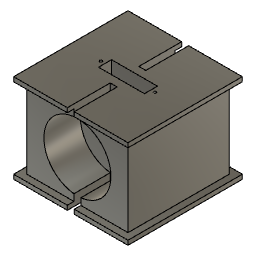
TWO MAG BODY 3x1.5 v01 (Autodesk Fusion 360 design; units mm, degrees)
Autodesk Fusion 360 part; units mm, degrees
note: some values were not read from the file. Set by a fixed rule: which sketch regions a step uses.
sketch "Sketch1" plane through (0, 0, 0) normal (0, 0, 1) x (1, 0, 0)
  line L0 (-30.48, 114.973) -> (86.36, 114.973)
  line L1 (86.36, 114.973) -> (86.36, -1.867)
  line L2 (86.36, -1.867) -> (-30.48, -1.867)
  line L3 (-30.48, -1.867) -> (-30.48, 114.973)
  line L4 (1.4449, 64.0587) -> (54.4449, 64.0587)
  line L5 (54.4449, 64.0587) -> (54.4449, 49.0587)
  line L6 (54.4449, 49.0587) -> (1.4449, 49.0587)
  line L7 (1.4449, 49.0587) -> (1.4449, 64.0587)
  line L8 (23.9405, 114.973) -> (31.9405, 114.973)
  line L9 (31.9405, 114.973) -> (31.9405, 73.063)
  line L10 (31.9405, 73.063) -> (23.9405, 73.063)
  line L11 (23.9405, 73.063) -> (23.9405, 114.973)
  line L12 (23.9405, -1.867) -> (31.9405, -1.867)
  line L13 (31.9405, -1.867) -> (31.9405, 40.043)
  line L14 (31.9405, 40.043) -> (23.9405, 40.043)
  line L15 (23.9405, 40.043) -> (23.9405, -1.867)
  dimension "d1" = 116.84
  dimension "d2" = 116.84
  dimension "d3" = 15
  dimension "d4" = 53
  dimension "d5" = 31.9151
  dimension "d8" = 50.9143
  dimension "d9" = 8
  dimension "d10" = 54.4195
  dimension "d11" = 41.91
  dimension "d12" = 41.91
  dimension "d13" = 54.4195
  dimension "d14" = 8
  constraint horizontal L0
  constraint vertical L1
  constraint horizontal L2
  constraint vertical L3
  constraint horizontal L4
  constraint vertical L5
  constraint horizontal L6
  constraint vertical L7
  constraint horizontal L8
  constraint vertical L9
  constraint horizontal L10
  constraint vertical L11
  constraint coincident L0 L8.start
  constraint horizontal L12
  constraint vertical L13
  constraint horizontal L14
  constraint vertical L15
  constraint coincident L2 L12.start
  measures "d1" distance of L0.end L1.end
  measures "d2" distance of L0.start L0.end
  measures "d3" distance of L4.end L5.end
  measures "d4" distance of L5.end L6.end
  measures "d5" distance of L1 L5
  measures "d8" distance of L0 L4
  measures "d9" distance of L13 L15
  measures "d10" distance of L1 L13
  measures "d11" distance of L12.end L13.end
  measures "d12" distance of L8.end L9.end
  measures "d13" distance of L1 L9
  measures "d14" distance of L9.end L10.end
extrude "Extrude1" add sketch "Sketch1" along normal blind 102.616 contours L0 L1 L2 L3 L9 L10 L11 L13 L14 L15
sketch "Sketch2" plane through (0, -1.867, 0) normal (0, -1, 0) x (1, 0, 0)
  line L0 (-30.48, 0) -> (23.9405, 0)
  line L1 (23.9405, 0) -> (23.9405, 102.616)
  line L2 (23.9405, 102.616) -> (-30.48, 102.616)
  line L3 (-30.48, 102.616) -> (-30.48, 0)
  circle A0 centre (27.94, 51.308) radius 38.735
  dimension "d17" = 77.47
  dimension "d18" = 51.308
  dimension "d19" = 58.42
  measures "d17" diameter of A0
  measures "d18" distance of L2 A0.centre
  measures "d19" distance of L3 A0.centre
extrude "Extrude2" cut sketch "Sketch2" against normal blind 42.037 contours L1 A0 | L1 A0
sketch "Sketch3" plane through (0, 114.973, 0) normal (0, 1, 0) x (-1, 0, 0)
  line L0 (-23.9405, 0) -> (30.48, 0)
  line L1 (30.48, 0) -> (30.48, 102.616)
  line L2 (30.48, 102.616) -> (-23.9405, 102.616)
  line L3 (-23.9405, 102.616) -> (-23.9405, 0)
  circle A0 centre (-27.94, 51.308) radius 38.735
  dimension "d22" = 77.47
  dimension "d23" = 58.42
  dimension "d24" = 51.308
  measures "d22" diameter of A0
  measures "d23" distance of L1 A0.centre
  measures "d24" distance of L2 A0.centre
extrude "Extrude3" cut sketch "Sketch3" against normal blind 42.037 contours L3 A0 | L3 A0
sketch "Sketch5" plane through (0, -1.867, 0) normal (0, -1, 0) x (1, 0, 0)
  arc A0 (31.9405, 12.7801) -> (31.9405, 89.8359) centre (27.94, 51.308) ccw
  line L0 (31.9405, 12.7801) -> (31.9405, 0)
  line L1 (31.9405, 0) -> (86.36, 0)
  line L2 (86.36, 0) -> (86.36, 102.616)
  line L3 (86.36, 102.616) -> (31.9405, 102.616)
  line L4 (31.9405, 102.616) -> (31.9405, 89.8359)
  line L5 (86.36, 102.616) -> (86.36, 97.536)
  line L6 (-30.48, 97.536) -> (-30.48, 102.616)
  line L7 (-30.48, 5.08) -> (-30.48, 0)
  line L8 (86.36, 0) -> (86.36, 5.08)
  line L9 (31.9405, 102.616) -> (31.9405, 97.536)
  line L10 (23.9405, 102.616) -> (23.9405, 97.536)
  line L11 (23.9405, 89.836) -> (23.9405, 102.616)
  line L12 (23.9405, 5.08) -> (23.9405, 0)
  line L13 (31.9405, 5.08) -> (31.9405, 0)
  line L14 (86.36, 97.536) -> (31.9405, 97.536)
  line L15 (23.9405, 97.536) -> (-30.48, 97.536)
  line L16 (-30.48, 102.616) -> (23.9405, 102.616)
  line L17 (31.9405, 102.616) -> (86.36, 102.616)
  line L18 (86.36, 5.08) -> (31.9405, 5.08)
  line L19 (23.9405, 5.08) -> (-30.48, 5.08)
  line L20 (-30.48, 0) -> (23.9405, 0)
  line L21 (31.9405, 0) -> (86.36, 0)
  line L22 (-30.48, 102.616) -> (23.9405, 102.616)
  dimension "d71" = 5.08
  constraint horizontal L16
  constraint vertical L5
  constraint horizontal L14
  constraint vertical L6
  constraint coincident L2 L5.end
  constraint coincident L3.end L16
  constraint coincident L4 L3.end
  constraint coincident L4 L9.end
  constraint coincident L10.end L14
  constraint perpendicular L10 L14
  constraint coincident L10.start L11
  constraint coincident L12.start L18
  constraint perpendicular L12 L20
  constraint coincident L0 L13.start
  constraint coincident L0 L1.start
  constraint coincident L0.end L20
  constraint collinear L14 L15
  constraint collinear L16 L17
  constraint collinear L18 L19
  constraint collinear L20 L21
  constraint coincident L10.start L22
  constraint coincident L0.end L1.start
  measures "d71" distance of L15 L16
extrude "Extrude5" add sketch "Sketch5" along normal blind 7.62 contours L0 L1 L2 L8 L13 L18 L21 | L2 L3 L4 L5 L9 L14 L17 | L6 L10 L11 L15 L16 L22 | L7 L12 L19 L20
sketch "Sketch6" plane through (86.36, 0, 0) normal (1, 0, 0) x (0, 1, 0)
  line L0 (-1.867, 0) -> (114.973, 0)
  line L1 (114.973, 0) -> (114.973, 102.616)
  line L2 (114.973, 102.616) -> (-9.487, 102.616)
  line L3 (-1.867, 97.536) -> (-1.867, 5.08)
  line L4 (-9.487, 102.616) -> (-9.487, 97.536)
  line L5 (-9.487, 97.536) -> (-1.867, 97.536)
  line L6 (-9.487, 102.616) -> (114.973, 102.616)
  line L7 (114.973, 102.616) -> (114.973, 97.536)
  line L8 (114.973, 97.536) -> (-9.487, 97.536)
  line L9 (-9.487, 97.536) -> (-9.487, 102.616)
  line L10 (-9.487, 5.08) -> (114.973, 5.08)
  line L11 (114.973, 5.08) -> (114.973, 0)
  line L12 (114.973, 0) -> (-9.487, 0)
  line L13 (-9.487, 0) -> (-9.487, 5.08)
  line L14 (-1.867, 5.08) -> (-9.487, 5.08)
  line L15 (-9.487, 5.08) -> (-9.487, 0)
  line L16 (-9.487, 0) -> (-1.867, 0)
  dimension "d54" = 5.08
  dimension "d55" = 5.08
  constraint horizontal L6
  constraint vertical L7
  constraint horizontal L8
  constraint vertical L9
  constraint coincident L1 L7.end
  constraint coincident L2.end L4.start
  constraint horizontal L10
  constraint vertical L11
  constraint horizontal L12
  constraint vertical L13
  constraint coincident L1 L0.end
  constraint coincident L12.end L13.start
  measures "d54" distance of L2.end L4.end
  measures "d55" distance of L10.start L12.end
extrude "Extrude6" add sketch "Sketch6" along normal blind 7.62 contours L0 L1 L10 L11 L12 L13 L14 L15 L16 | L1 L2 L4 L5 L6 L7 L8 L9
sketch "Sketch7" plane through (0, 114.973, 0) normal (0, 1, 0) x (-1, 0, 0)
  arc A0 (-31.9405, 89.8359) -> (-31.9405, 12.7801) centre (-27.94, 51.308) ccw
  line L0 (-31.9405, 89.8359) -> (-31.9405, 102.616)
  line L1 (-31.9405, 102.616) -> (-93.98, 102.616)
  line L2 (-93.98, 102.616) -> (-93.98, 97.536)
  line L3 (-93.98, 97.536) -> (-86.36, 97.536)
  line L4 (-86.36, 97.536) -> (-86.36, 5.08)
  line L5 (-86.36, 5.08) -> (-93.98, 5.08)
  line L6 (-93.98, 5.08) -> (-93.98, 0)
  line L7 (-93.98, 0) -> (-31.9405, 0)
  line L8 (-31.9405, 0) -> (-31.9405, 12.7801)
  line L9 (30.48, 102.616) -> (30.48, 97.536)
  line L10 (-93.98, 97.536) -> (-93.98, 102.616)
  line L11 (30.48, 0) -> (30.48, 102.616)
  line L12 (30.48, 5.08) -> (30.48, 0)
  line L13 (-93.98, 0) -> (-93.98, 5.08)
  line L14 (-23.9405, 102.616) -> (-23.9405, 97.536)
  line L15 (-23.9405, 89.836) -> (-23.9405, 102.616)
  line L16 (-31.9405, 102.616) -> (-31.9405, 97.536)
  line L17 (-31.9405, 5.08) -> (-31.9405, 0)
  line L18 (-23.9405, 5.08) -> (-23.9405, 0)
  line L19 (-23.9405, 0) -> (-23.9405, 12.78)
  line L20 (-93.98, 5.08) -> (-31.9405, 5.08)
  line L21 (-23.9405, 5.08) -> (30.48, 5.08)
  line L22 (30.48, 0) -> (-23.9405, 0)
  line L23 (-31.9405, 0) -> (-93.98, 0)
  line L24 (-93.98, 102.616) -> (-31.9405, 102.616)
  line L25 (-23.9405, 102.616) -> (30.48, 102.616)
  line L26 (30.48, 97.536) -> (-23.9405, 97.536)
  line L27 (-31.9405, 97.536) -> (-93.98, 97.536)
  dimension "d58" = 5.08
  dimension "d59" = 5.08
  constraint horizontal L24
  constraint vertical L9
  constraint horizontal L26
  constraint vertical L10
  constraint coincident L1.end L2.start
  constraint coincident L9.end L11
  constraint horizontal L20
  constraint vertical L12
  constraint horizontal L22
  constraint vertical L13
  constraint coincident L11 L12.end
  constraint coincident L5.end L6.start
  constraint coincident L14.start L24
  constraint perpendicular L14 L26
  constraint coincident L14.start L15
  constraint coincident L0 L1.start
  constraint coincident L16.end L26
  constraint coincident L0 L16.end
  constraint coincident L8 L17.start
  constraint coincident L7.end L22
  constraint coincident L8 L7.end
  constraint coincident L18.start L20
  constraint perpendicular L18 L22
  constraint coincident L18.start L19
  constraint collinear L20 L21
  constraint collinear L22 L23
  constraint collinear L24 L25
  constraint collinear L26 L27
  measures "d58" distance of L1.end L2.end
  measures "d59" distance of L5.end L6.end
extrude "Extrude7" add sketch "Sketch7" along normal blind 7.62 contours L0 L1 L2 L3 L10 L16 L24 L27 | L5 L6 L7 L8 L13 L17 L20 L23 | L9 L11 L14 L15 L25 L26 | L11 L12 L18 L19 L21 L22
sketch "Sketch8" plane through (-30.48, 0, 0) normal (-1, 0, 0) x (0, -1, 0)
  line L0 (-122.593, 0) -> (1.867, 0)
  line L1 (1.867, 5.08) -> (1.867, 97.536)
  line L2 (1.867, 97.536) -> (9.487, 97.536)
  line L3 (9.487, 0) -> (9.487, 5.08)
  line L4 (9.487, 102.616) -> (-122.593, 102.616)
  line L5 (-122.593, 102.616) -> (-122.593, 97.536)
  line L6 (-122.593, 97.536) -> (-114.973, 97.536)
  line L7 (-114.973, 97.536) -> (-114.973, 5.08)
  line L8 (-114.973, 5.08) -> (-122.593, 5.08)
  line L9 (-122.593, 5.08) -> (-122.593, 0)
  line L10 (1.867, 0) -> (9.487, 0)
  line L11 (9.487, 5.08) -> (1.867, 5.08)
  line L12 (9.487, 97.536) -> (9.487, 102.616)
  line L13 (-122.593, 102.616) -> (9.487, 102.616)
  line L14 (9.487, 102.616) -> (9.487, 97.536)
  line L15 (9.487, 97.536) -> (-122.593, 97.536)
  line L16 (-122.593, 97.536) -> (-122.593, 102.616)
  line L17 (-122.593, 5.08) -> (9.487, 5.08)
  line L18 (9.487, 5.08) -> (9.487, 0)
  line L19 (9.487, 0) -> (-122.593, 0)
  line L20 (-122.593, 0) -> (-122.593, 5.08)
  constraint horizontal L13
  constraint vertical L14
  constraint horizontal L15
  constraint vertical L16
  constraint coincident L2.end L12.start
  constraint coincident L4.end L5.start
  constraint horizontal L17
  constraint vertical L18
  constraint horizontal L19
  constraint vertical L20
  constraint coincident L3.start L10.end
  constraint coincident L8.end L9.start
sketch "Sketch9" plane through (0, 0, 102.616) normal (0, 0, 1) x (-1, 0, 0)
  line L0 (-54.4449, -49.0587) -> (-1.4449, -49.0587)
  line L1 (-1.4449, -49.0587) -> (-1.4449, -64.0587)
  line L2 (-1.4449, -64.0587) -> (-54.4449, -64.0587)
  line L3 (-54.4449, -64.0587) -> (-54.4449, -49.0587)
  line L4 (-31.9405, -122.593) -> (-31.9405, -73.063)
  line L5 (-31.9405, -73.063) -> (-23.9405, -73.063)
  line L6 (-23.9405, -73.063) -> (-23.9405, -122.593)
  line L7 (-23.9405, 9.487) -> (-23.9405, -40.043)
  line L8 (-23.9405, -40.043) -> (-31.9405, -40.043)
  line L9 (-31.9405, -40.043) -> (-31.9405, 9.487)
  circle A0 centre (3.2541, -56.5587) radius 1.5
  circle A1 centre (-59.1459, -56.5587) radius 1.5
  line L10 (-23.9405, -122.593) -> (30.48, -122.593)
  line L11 (30.48, 9.487) -> (-23.9405, 9.487)
  line L12 (-31.9405, 9.487) -> (-93.98, 9.487)
  line L13 (-93.98, 9.487) -> (-93.98, -122.593)
  line L14 (-93.98, -122.593) -> (-31.9405, -122.593)
  line L15 (30.48, -122.593) -> (30.48, 9.487)
  dimension "d64" = 3
  dimension "d65" = 3
  dimension "d66" = 62.4
  dimension "d67" = 4.699
  dimension "d68" = 7.5
  measures "d64" diameter of A0
  measures "d65" diameter of A1
  measures "d66" distance of A0.centre A1.centre
  measures "d67" distance of L1 A0.centre
  measures "d68" distance of L2 A1.centre
extrude "Extrude9" cut sketch "Sketch9" against normal blind 12.7 contours A0 | A1
extrude "Extrude10" add sketch "Sketch8" along normal blind 7.62 contours L0 L3 L8 L9 L10 L11 L17 L18 L19 L20 | L2 L4 L5 L6 L12 L13 L14 L15 L16
